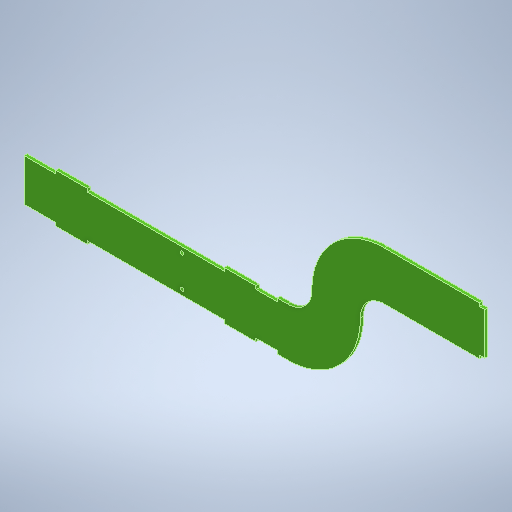
# Autodesk Inventor part: Starting Path
Saved by Autodesk Inventor 2025.4 (Build 294407000, 407)
## iProperties
Created: 2026-05-18
Part Number: Starting Path
Material: Generic
Document SubType Name: Sheet Metal
Designer: lenovo
Density: 1 g/cm^3
Sheet Metal Rule: Default_mm
Appearance: Default(1)
Author: lenovo
Autodesk Inventor part; units mm, degrees
ref_plane "YZ Plane" through (0, 0, 0) normal (1, 0, 0) x (0, 1, 0)
ref_plane "XZ Plane" through (0, 0, 0) normal (0, 1, 0) x (-1, 0, 0)
ref_plane "XY Plane" through (0, 0, 0) normal (0, 0, 1) x (1, 0, 0)
sketch "Sketch1" plane through (0, 0, 0) normal (0, 0, 1) x (1, 0, 0)
  line L0 (-125, -20) -> (125, -20)
  line L1 (125, -20) -> (125, 20)
  line L2 (125, 20) -> (-125, 20)
  line L3 (-125, 20) -> (-125, -20)
  line L4 (-125, -20) -> (125, 20) construction
  line L5 (125, -20) -> (-125, 20) construction
  line L6 (125, 20) -> (115, 20)
  line L7 (115, 20) -> (115, 23)
  line L8 (115, 23) -> (125, 23)
  line L9 (125, 23) -> (125, 20)
  arc A0 (125, 20) -> (151, 46) centre (125, 46) ccw
  arc A1 (125, 23) -> (148, 46) centre (125, 46) ccw
  line L10 (151, 46) -> (148, 46)
  line L11 (125, -20) -> (115, -20)
  line L12 (115, -20) -> (115, -23)
  line L13 (115, -23) -> (125, -23)
  line L14 (125, -23) -> (125, -20)
  arc A2 (125, -20) -> (191, 46) centre (125, 46) ccw
  arc A3 (125, -23) -> (194, 46) centre (125, 46) ccw
  line L15 (194, 46) -> (191, 46)
  line L16 (151, 46) -> (191, 46)
  arc A4 (217, 115) -> (148, 46) centre (217, 46) ccw
  arc A5 (217, 69) -> (194, 46) centre (217, 46) ccw
  arc A6 (217, 72) -> (191, 46) centre (217, 46) ccw
  arc A7 (217, 112) -> (151, 46) centre (217, 46) ccw
  line L17 (217, 115) -> (217, 69)
  line L18 (217, 112) -> (312, 112)
  line L19 (312, 112) -> (312, 72)
  line L20 (312, 72) -> (217, 72)
  line L21 (217, 72) -> (217, 112)
  line L22 (-95, -20) -> (-65, -20)
  line L23 (-65, -20) -> (-65, -23)
  line L24 (-65, -23) -> (-95, -23)
  line L25 (-95, -23) -> (-95, -20)
  line L26 (95, -20) -> (65, -20)
  line L27 (65, -20) -> (65, -23)
  line L28 (65, -23) -> (95, -23)
  line L29 (95, -23) -> (95, -20)
  line L30 (-125, 0) -> (125, 0)
  line L31 (-95, 20) -> (-65, 20)
  line L32 (-65, 20) -> (-65, 23)
  line L33 (-65, 23) -> (-95, 23)
  line L34 (-95, 23) -> (-95, 20)
  line L35 (95, 20) -> (65, 20)
  line L36 (65, 20) -> (65, 23)
  line L37 (65, 23) -> (95, 23)
  line L38 (95, 23) -> (95, 20)
  line L39 (217, 112) -> (307, 112)
  line L40 (307, 112) -> (307, 115)
  line L41 (307, 115) -> (217, 115)
  line L42 (217, 115) -> (217, 112)
  line L43 (312, 72) -> (217, 72)
  line L44 (217, 72) -> (217, 69)
  line L45 (217, 69) -> (307, 69)
  line L46 (307, 69) -> (307, 72)
  line L47 (307, 72) -> (217, 72)
  line L48 (217, 72) -> (217, 69)
  point P0 (0, 0)
  point P1 (125, 21.5)
  point P2 (149.5, 46)
  point P3 (125, 23)
  point P4 (115, 20)
  point P5 (115, -20)
  point P6 (125, -23)
  point P7 (192.5, 46)
  point P8 (217, 72)
  point P9 (217, 115)
  point P10 (307, 112)
  point P11 (307, 72)
  dimension "d0" = 250
  dimension "d1" = 40
  dimension "d2" = 10
  dimension "d3" = 3
  dimension "d5" = 26
  dimension "d6" = 3
  dimension "d7" = 10
  dimension "d8" = 3
  dimension "d10" = 3
  dimension "d12" = 3
  dimension "d13" = 3
  dimension "d14" = 95
  dimension "d15" = 40
  dimension "d29" = 30
  dimension "d30" = 3
  dimension "d31" = 30
  dimension "d32" = 30
  dimension "d33" = 3
  dimension "d34" = 20
  dimension "d35" = 90
  dimension "d36" = 3
  dimension "d39" = 90
  dimension "d40" = 3
  measures "d0" distance of L2.end L1.end
  measures "d1" distance of L1.end L0.end
  measures "d2" distance of L7.end L8.end
  measures "d3" distance of L6.end L7.end
  measures "d5" radius of A0
  measures "d6" radial gap between concentric circles of A0 A1
  measures "d7" distance of L13.end L12.end
  measures "d8" distance of L12.end L11.end
  measures "d10" radial gap between concentric circles of A2 A3
  measures "d12" radial gap between concentric circles of A5 A6
  measures "d13" radial gap between concentric circles of A4 A7
  measures "d14" distance of L19.end L20.end
  measures "d15" distance of L18.end L19.end
  measures "d29" distance of L23.end L24.end
  measures "d30" distance of L22.end L23.end
  measures "d31" distance between parallel lines of L3 L25
  measures "d32" distance of L28.end L27.end
  measures "d33" distance of L27.end L26.end
  measures "d34" distance between parallel lines of L29 L12
  measures "d35" distance of L41.end L40.end
  measures "d36" distance of L40.end L39.end
  measures "d39" distance of L46.end L47.end
  measures "d40" distance between parallel lines of L47 L45
extrude "Plate1" add sketch "Sketch1" along normal blind 3
sketch "Sketch2" plane through (0, 0, 3) normal (0, 0, 1) x (1, 0, 0)
  circle A0 centre (25, 15) radius 1.6
  line L0 (0, 0) -> (25, 0)
  circle A1 centre (25, -15) radius 1.6
  dimension "d41" = 3.2
  dimension "d43" = 30
  dimension "d44" = 25
  constraints: 2 centre point, 2 end point, 1 horizontal, 1 symmetric about line, 1 vertical alignment, 1 other
  measures "d41" diameter of A0
  measures "d43" diameter of A0.centre L0
  measures "d44" horizontal distance of L0.start A0.centre
extrude "Cut1" cut sketch "Sketch2" against normal blind 3
equation "\"d7\" = d2"
equation "\"d39\" = d35"
equation "\"d40\" = d36"
equation "\"d45\" = Thickness"
equation "\"d11\" = Thickness"
equation "\"BendRadius\" = Thickness"
equation "\"BendReliefWidth\" = Thickness"
equation "\"BendReliefDepth\" = 0.5 * Thickness"
equation "\"CornerReliefSize\" = 4 * Thickness"
equation "\"MinimumRemnant\" = 2 * Thickness"
equation "\"TransitionRadius\" = BendRadius"
equation "\"JacobiRadiusSize\" = BendRadius"
equation "\"GapSize\" = Thickness"
equation "\"Thickness\" = 3"
body "Solid1"
